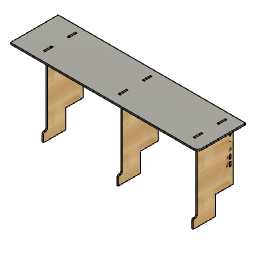
Overall_proto_v3 (Autodesk Fusion 360 design; units mm, degrees)
Autodesk Fusion 360 part; units mm, degrees
sketch "Sketch1" plane through (0, 0, 0) normal (0, 0, 1) x (1, 0, 0)
  line L0 (-1175, 300) -> (1175, 300)
  line L1 (1175, 300) -> (1175, -300)
  line L2 (1175, -300) -> (-1175, -300)
  line L3 (-1175, -300) -> (-1175, 300)
  line L4 (-1175, 300) -> (1175, -300) construction
  line L5 (1175, 300) -> (-1175, -300) construction
  dimension "d5" = 2350
  dimension "d6" = 600
  constraint perpendicular L0 L1
  constraint parallel L0 L2
  constraint parallel L1 L3
  constraint horizontal L0
  constraint coincident L4 origin
  constraint coincident L5 origin
  measures "d5" distance of L1.end L2.end
  measures "d6" distance of L0.end L1.end
extrude "Extrude1" add sketch "Sketch1" along normal blind 18 makes body 1
fillet "Fillet1" radius 50 1 edges at (1175, -300, 9) on bodies 1
sketch "Sketch2" plane through (0, 0, 18) normal (0, 0, 1) x (-1, 0, 0)
  arc A0 (-1125, 300) -> (-1175, 250) centre (-1125, 250) ccw
  line L0 (-1175, 250) -> (-1175, -300)
  line L1 (-1175, -300) -> (1175, -300)
  line L2 (1175, -300) -> (1175, 300)
  line L3 (1175, 300) -> (-1125, 300)
  line L4 (-61, -120) -> (-79, -120)
  line L5 (-79, -120) -> (-79, -220)
  line L6 (-79, -220) -> (-61, -220)
  line L7 (-61, -220) -> (-61, -120)
  line L8 (-61, -120) -> (-79, -220) construction
  line L9 (-79, -120) -> (-61, -220) construction
  point P0 (-70, -170)
  dimension "d10" = 18
  dimension "d11" = 100
  dimension "d12" = 80
  dimension "d23" = 70
  constraint perpendicular L4 L5
  constraint parallel L4 L6
  constraint parallel L5 L7
  constraint horizontal L4
  constraint coincident L8 P0
  constraint coincident L9 P0
  measures "d10" distance of L5.end L6.end
  measures "d11" distance of L4.end L5.end
  measures "d12" distance of L1 L6.end
  measures "d23" horizontal distance of origin P0
extrude "Extrude2" cut sketch "Sketch2" against normal blind 18 contours L4 L5 L6 L7 bodies 1
sketch "Sketch3" plane through (0, 0, 18) normal (0, 0, 1) x (-1, 0, 0)
  line L0 (-79, -120) -> (-61, -120)
  line L1 (-61, -120) -> (-61, -220)
  line L2 (-61, -220) -> (-79, -220)
  line L3 (-79, -220) -> (-79, -120)
  arc A0 (-1125, 300) -> (-1175, 250) centre (-1125, 250) ccw
  line L4 (-1175, 250) -> (-1175, -300)
  line L5 (-1175, -300) -> (1175, -300)
  line L6 (1175, -300) -> (1175, 300)
  line L7 (1175, 300) -> (-1125, 300)
  circle A1 centre (-61, -216.9375) radius 3.0625
  line L8 (-61, -170) -> (-79, -170) construction
  line L9 (-70, -220) -> (-70, -120) construction
  circle A2 centre (-79, -216.9375) radius 3.0625
  line L10 (-61, -120) -> (-79, -120)
  circle A3 centre (-61, -123.0625) radius 3.0625
  circle A4 centre (-79, -123.0625) radius 3.0625
  point P0 (-79, -220)
  point P1 (-79, -120)
  point P2 (-70, -120)
  dimension "d16" = 6.125
  constraint coincident L1 A1.centre
  constraint tangent L2 A1
  constraint midpoint L1 L8.start
  constraint midpoint L3 L8.end
  constraint midpoint L2 L9.start
  constraint midpoint L0 P2
  constraint symmetric L1.end L9 P0
  constraint symmetric A1 L9 A2
  constraint symmetric L1.end L8 L0.end
  constraint symmetric P0 L8 P1
  constraint symmetric A1 L8 A3
  constraint symmetric L8 L9.start P2
  constraint symmetric L8 P0 P1
  constraint symmetric L8 A2 A4
  measures "d16" diameter of A1
extrude "Extrude3" cut sketch "Sketch3" against normal blind 18 contours L3 A4 | L1 A3 | L3 A2 | L1 A1 picked at (-80.1701, -122.9976) picked at (-58.9279, -123.5072) picked at (-80.1701, -217.0024) picked at (-60.4481, -216.0787) bodies 1
pattern_linear "R-Pattern1" count 3 spacing 940 along (1, 0, 0) both ways count 2 spacing 300 along (0, -1, 0) of "Extrude2", "Extrude3"
sketch "Sketch4" plane through (0, 0, 0) normal (1, 0, 0) x (0, 1, 0)
  line L0 (300, -44.3727) -> (-200, -44.3727)
  line L1 (-200, -44.3727) -> (-200, -1008.3727)
  line L2 (-200, -1008.3727) -> (300, -1008.3727)
  line L3 (300, -1008.3727) -> (300, -44.3727)
  line L4 (300, -1008.3727) -> (79, -1008.3727)
  line L5 (79, -1008.3727) -> (79, -768.3727)
  line L6 (79, -768.3727) -> (300, -768.3727)
  line L7 (300, -768.3727) -> (300, -1008.3727)
  line L8 (220, -44.3727) -> (120, -44.3727)
  line L9 (120, -44.3727) -> (120, -26.3727)
  line L10 (120, -26.3727) -> (220, -26.3727)
  line L11 (220, -26.3727) -> (220, -44.3727)
  line L12 (-180, -26.3727) -> (-80, -26.3727)
  line L13 (-180, -44.3727) -> (-180, -26.3727)
  line L14 (-80, -44.3727) -> (-180, -44.3727)
  line L15 (-80, -26.3727) -> (-80, -44.3727)
  dimension "d24" = 964
  dimension "d25" = 500
  dimension "d29" = 240
  dimension "d30" = 221
  dimension "d31" = 100
  dimension "d32" = 18
  dimension "d35" = 80
  dimension "d38" = 300
  dimension "d39" = 0
  constraint horizontal L0
  constraint vertical L1
  constraint horizontal L2
  constraint vertical L3
  constraint horizontal L4
  constraint vertical L5
  constraint horizontal L6
  constraint vertical L7
  constraint horizontal L8
  constraint vertical L9
  constraint horizontal L10
  constraint vertical L11
  constraint coincident L0 L8.start
  measures "d24" distance of L0.start L2.end
  measures "d25" distance of L0.start L0.end
  measures "d29" distance of L2.end L6.end
  measures "d30" distance of L2.end L4.end
  measures "d31" distance of L8.start L8.end
  measures "d32" distance of L8.start L10.end
  measures "d35" distance of L3 L8.start
extrude "Extrude4" add sketch "Sketch4" along normal blind 18 separate body contours L0 L1 L2 L3 L5 L6 L8 L14 | L0 L8 L9 L10 L11 | L0 L12 L13 L14 L15 makes body 2
sketch "Sketch5" plane through (0, 0, 0) normal (-1, 0, 0) x (0, -1, 0)
  line L0 (200, -44.3727) -> (180, -44.3727)
  line L1 (180, -44.3727) -> (180, -26.3727)
  line L2 (180, -26.3727) -> (80, -26.3727)
  line L3 (80, -26.3727) -> (80, -44.3727)
  line L4 (80, -44.3727) -> (-120, -44.3727)
  line L5 (-120, -44.3727) -> (-120, -26.3727)
  line L6 (-120, -26.3727) -> (-220, -26.3727)
  line L7 (-220, -26.3727) -> (-220, -44.3727)
  line L8 (-220, -44.3727) -> (-300, -44.3727)
  line L9 (-300, -44.3727) -> (-300, -768.3727)
  line L10 (-300, -768.3727) -> (-79, -768.3727)
  line L11 (-79, -768.3727) -> (-79, -1008.3727)
  line L12 (-79, -1008.3727) -> (200, -1008.3727)
  line L13 (200, -1008.3727) -> (200, -44.3727)
  circle A0 centre (-223.0625, -44.3727) radius 3.0625
  circle A1 centre (-116.9375, -44.3727) radius 3.0625
  circle A2 centre (183.0625, -44.3727) radius 3.0625
  circle A3 centre (76.9375, -44.3727) radius 3.0625
  point P0 (-113.875, -44.3727)
  point P1 (186.125, -44.3727)
  point P2 (180, -44.3727)
  point P3 (80, -44.3727)
  dimension "d42" = 6.125
  dimension "d45" = 106.125
  dimension "d46" = 0
  dimension "d49" = 300
  dimension "d50" = 0
  constraint coincident L7.end A0
  measures "d42" diameter of A0
extrude "Extrude5" cut sketch "Sketch5" against normal blind 18 contours L0 A2 | L4 A3 | L8 A0 | L4 A1 picked at (183.1388, -45.3906) picked at (76.8612, -45.3906) picked at (-223.1388, -45.3906) picked at (-117.0138, -45.3906) bodies 2
fillet "Fillet2" radius 6.125 4 edges at (9, 220, -26.3727) (9, 120, -26.3727) (9, -180, -26.3727) (9, -80, -26.3727) on bodies 2
sketch "Sketch6" plane through (0, 0, 0) normal (-1, 0, 0) x (0, -1, 0)
  arc A0 (86.125, -26.3727) -> (80, -32.4977) centre (86.125, -32.4977) ccw
  line L0 (80, -32.4977) -> (80, -44.3727)
  arc A1 (73.875, -44.3727) -> (80, -44.3727) centre (76.9375, -44.3727) ccw
  line L1 (73.875, -44.3727) -> (-113.875, -44.3727)
  arc A2 (-120, -44.3727) -> (-113.875, -44.3727) centre (-116.9375, -44.3727) ccw
  line L2 (-120, -44.3727) -> (-120, -32.4977)
  arc A3 (-120, -32.4977) -> (-126.125, -26.3727) centre (-126.125, -32.4977) ccw
  line L3 (-126.125, -26.3727) -> (-213.875, -26.3727)
  arc A4 (-213.875, -26.3727) -> (-220, -32.4977) centre (-213.875, -32.4977) ccw
  line L4 (-220, -32.4977) -> (-220, -44.3727)
  arc A5 (-226.125, -44.3727) -> (-220, -44.3727) centre (-223.0625, -44.3727) ccw
  line L5 (-226.125, -44.3727) -> (-300, -44.3727)
  line L6 (-300, -44.3727) -> (-300, -768.3727)
  line L7 (-300, -768.3727) -> (-79, -768.3727)
  line L8 (-79, -768.3727) -> (-79, -1008.3727)
  line L9 (-79, -1008.3727) -> (200, -1008.3727)
  line L10 (200, -1008.3727) -> (200, -44.3727)
  line L11 (200, -44.3727) -> (186.125, -44.3727)
  arc A6 (180, -44.3727) -> (186.125, -44.3727) centre (183.0625, -44.3727) ccw
  line L12 (180, -44.3727) -> (180, -32.4977)
  arc A7 (180, -32.4977) -> (173.875, -26.3727) centre (173.875, -32.4977) ccw
  line L13 (173.875, -26.3727) -> (86.125, -26.3727)
  circle A8 centre (-79, -771.4352) radius 3.0625
  dimension "d54" = 6.125
  constraint coincident L7.end A8
  measures "d54" diameter of A8
extrude "Extrude6" cut sketch "Sketch6" against normal blind 18 contours L8 A8 picked at (-77.1359, -770.6096) bodies 2
sketch "Sketch7" plane through (18, 0, 0) normal (1, 0, 0) x (0, 1, 0)
  arc A0 (79, -768.3727) -> (79, -774.4977) centre (79, -771.4352) ccw
  line L0 (79, -768.3727) -> (300, -768.3727)
  line L1 (300, -768.3727) -> (300, -44.3727)
  line L2 (300, -44.3727) -> (226.125, -44.3727)
  arc A1 (220, -44.3727) -> (226.125, -44.3727) centre (223.0625, -44.3727) ccw
  line L3 (220, -44.3727) -> (220, -32.4977)
  arc A2 (220, -32.4977) -> (213.875, -26.3727) centre (213.875, -32.4977) ccw
  line L4 (213.875, -26.3727) -> (126.125, -26.3727)
  arc A3 (126.125, -26.3727) -> (120, -32.4977) centre (126.125, -32.4977) ccw
  line L5 (120, -32.4977) -> (120, -44.3727)
  arc A4 (113.875, -44.3727) -> (120, -44.3727) centre (116.9375, -44.3727) ccw
  line L6 (113.875, -44.3727) -> (-73.875, -44.3727)
  arc A5 (-80, -44.3727) -> (-73.875, -44.3727) centre (-76.9375, -44.3727) ccw
  line L7 (-80, -44.3727) -> (-80, -32.4977)
  arc A6 (-80, -32.4977) -> (-86.125, -26.3727) centre (-86.125, -32.4977) ccw
  line L8 (-86.125, -26.3727) -> (-173.875, -26.3727)
  arc A7 (-173.875, -26.3727) -> (-180, -32.4977) centre (-173.875, -32.4977) ccw
  line L9 (-180, -32.4977) -> (-180, -44.3727)
  arc A8 (-186.125, -44.3727) -> (-180, -44.3727) centre (-183.0625, -44.3727) ccw
  line L10 (-186.125, -44.3727) -> (-200, -44.3727)
  line L11 (-200, -44.3727) -> (-200, -1008.3727)
  line L12 (-200, -1008.3727) -> (79, -1008.3727)
  line L13 (79, -1008.3727) -> (79, -774.4977)
  line L14 (-200, -150) -> (-170, -150)
  line L15 (-150, -170) -> (-150, -880)
  line L16 (-170, -900) -> (-200, -900)
  line L17 (-200, -900) -> (-200, -150)
  arc A9 (-150, -170) -> (-170, -150) centre (-170, -170) ccw
  arc A10 (-170, -900) -> (-150, -880) centre (-170, -880) ccw
  dimension "d57" = 20
  constraint horizontal L14
  constraint vertical L15
  constraint horizontal L16
  constraint vertical L17
  constraint coincident L11 L14.start
  constraint tangent L14 A9
  constraint tangent L15 A9
  constraint tangent L15 A10
  constraint tangent L16 A10
  constraint equal A9 A10
  measures "d57" radius of A9
extrude "Extrude7" cut sketch "Sketch7" against normal blind 18 contours L11 L14 L15 L16 L17 A9 A10 bodies 2
sketch "Sketch8" plane through (18, 0, 0) normal (1, 0, 0) x (0, 1, 0)
  line L0 (-200, -150) -> (-170, -150)
  arc A0 (-150, -170) -> (-170, -150) centre (-170, -170) ccw
  line L1 (-150, -170) -> (-150, -880)
  arc A1 (-170, -900) -> (-150, -880) centre (-170, -880) ccw
  line L2 (-170, -900) -> (-200, -900)
  line L3 (-200, -900) -> (-200, -1008.3727)
  line L4 (-200, -1008.3727) -> (79, -1008.3727)
  line L5 (79, -1008.3727) -> (79, -774.4977)
  arc A2 (79, -768.3727) -> (79, -774.4977) centre (79, -771.4352) ccw
  line L6 (79, -768.3727) -> (300, -768.3727)
  line L7 (300, -768.3727) -> (300, -44.3727)
  line L8 (300, -44.3727) -> (226.125, -44.3727)
  arc A3 (220, -32.4977) -> (213.875, -26.3727) centre (213.875, -32.4977) ccw
  line L9 (213.875, -26.3727) -> (126.125, -26.3727)
  arc A4 (126.125, -26.3727) -> (120, -32.4977) centre (126.125, -32.4977) ccw
  line L10 (120, -32.4977) -> (120, -44.3727)
  arc A5 (113.875, -44.3727) -> (120, -44.3727) centre (116.9375, -44.3727) ccw
  line L11 (113.875, -44.3727) -> (-73.875, -44.3727)
  arc A6 (-80, -44.3727) -> (-73.875, -44.3727) centre (-76.9375, -44.3727) ccw
  line L12 (-80, -44.3727) -> (-80, -32.4977)
  arc A7 (-80, -32.4977) -> (-86.125, -26.3727) centre (-86.125, -32.4977) ccw
  line L13 (-86.125, -26.3727) -> (-173.875, -26.3727)
  arc A8 (-173.875, -26.3727) -> (-180, -32.4977) centre (-173.875, -32.4977) ccw
  line L14 (-180, -32.4977) -> (-180, -44.3727)
  arc A9 (-186.125, -44.3727) -> (-180, -44.3727) centre (-183.0625, -44.3727) ccw
  line L15 (-186.125, -44.3727) -> (-200, -44.3727)
  line L16 (-200, -44.3727) -> (-200, -150)
  line L17 (273, -94.3727) -> (273, -144.3727)
  circle A10 centre (258.0625, -144.3727) radius 3.0625
  line L18 (255, -94.3727) -> (273, -94.3727)
  line L19 (273, -144.3727) -> (255, -144.3727)
  line L20 (255, -144.3727) -> (255, -94.3727)
  circle A11 centre (269.9375, -144.3727) radius 3.0625
  circle A12 centre (269.9375, -94.3727) radius 3.0625
  circle A13 centre (258.0625, -94.3727) radius 3.0625
  line L21 (255, -427.706) -> (273, -427.706)
  line L22 (273, -427.706) -> (273, -477.706)
  circle A14 centre (269.9375, -477.706) radius 3.0625
  line L23 (255, -477.706) -> (255, -427.706)
  circle A15 centre (258.0625, -427.706) radius 3.0625
  circle A16 centre (258.0625, -477.706) radius 3.0625
  line L24 (273, -477.706) -> (255, -477.706)
  circle A17 centre (269.9375, -427.706) radius 3.0625
  line L25 (264, -144.3727) -> (264, -427.706) construction
  circle A18 centre (264, -286.0393) radius 2.5
  dimension "d78" = 18
  dimension "d79" = 6.125
  dimension "d80" = 27
  dimension "d81" = 50
  dimension "d84" = 0
  dimension "d85" = -333.3333
  dimension "d86" = 5
  constraint tangent L20 A13
  constraint tangent A10 L20
  constraint tangent L17 A12
  constraint tangent L17 A11
  constraint coincident L18 A13.centre
  constraint coincident L18 A12.centre
  constraint coincident A10.centre L19
  constraint coincident A11.centre L19
  constraint equal A12 A13
  constraint equal A10 A12
  constraint equal A10 A11
  constraint midpoint L19 L25.start
  constraint midpoint L21 L25.end
  constraint midpoint L25 A18.centre
  measures "d78" distance of L17 L20
  measures "d79" diameter of A13
  measures "d80" distance of L7 L17
  measures "d81" distance of L8 L18
  measures "d86" diameter of A18
extrude "Extrude8" cut sketch "Sketch8" against normal blind 18 bodies 2
pattern_linear "R-Pattern2" count 2 spacing 80 along (0, 0, -1) of "Extrude8"
fillet "Fillet3" radius 20 2 edges at (9, -200, -900) (9, -200, -150) on bodies 2
copy_body "Body->Comp1" bodies 1 removing the originals makes body 3 in component "btm_sheet"
copy_body "Body->Comp2" bodies 2 removing the originals makes body 4 in component "stand"
sketch "Sketch9" plane through (0, 0, 0) normal (0, 1, 0) x (1, 0, 0)
  line L0 (74.3329, 269.9769) -> (-901.6671, 269.9769)
  line L1 (-901.6671, 269.9769) -> (-901.6671, 653.3103)
  line L2 (-901.6671, 653.3103) -> (74.3329, 653.3103)
  line L3 (74.3329, 653.3103) -> (74.3329, 269.9769)
  line L4 (74.3329, 319.9769) -> (56.3329, 319.9769)
  line L5 (56.3329, 319.9769) -> (56.3329, 603.3103)
  line L6 (56.3329, 603.3103) -> (74.3329, 603.3103)
  line L7 (74.3329, 603.3103) -> (74.3329, 319.9769)
  circle A0 centre (56.3329, 323.0394) radius 3.0625
  circle A1 centre (56.3329, 600.2478) radius 3.0625
  line L8 (-413.6671, 269.9769) -> (-413.6671, 653.3103) construction
  line L9 (56.3329, 529.1436) -> (56.3329, 494.1436)
  circle A2 centre (-883.6671, 323.0394) radius 3.0625
  line L10 (-901.6671, 603.3103) -> (-901.6671, 319.9769)
  line L11 (-883.6671, 603.3103) -> (-901.6671, 603.3103)
  circle A3 centre (-883.6671, 600.2478) radius 3.0625
  line L12 (-883.6671, 319.9769) -> (-883.6671, 603.3103)
  line L13 (-901.6671, 319.9769) -> (-883.6671, 319.9769)
  line L14 (-883.6671, 529.1436) -> (-883.6671, 494.1436)
  point P0 (-3.6671, 511.6436)
  dimension "d122" = 976
  dimension "d123" = 383.3333
  dimension "d124" = 283.3333
  dimension "d125" = 18
  dimension "d126" = 6.125
  dimension "d127" = 6.125
  constraint horizontal L0
  constraint vertical L1
  constraint horizontal L2
  constraint vertical L3
  constraint horizontal L4
  constraint vertical L5
  constraint horizontal L6
  constraint coincident L3 L4.start
  constraint coincident L4.end A0
  constraint coincident L5.end A1
  constraint midpoint L0 L8.start
  constraint midpoint L2 L8.end
  constraint vertical L9
  constraint coincident L5 L9.end
  constraint symmetric L4.start L8 L10.end
  constraint symmetric L4.end L8 L12.start
  constraint symmetric L5.end L8 L11.start
  constraint symmetric L6.end L8 L10.start
  constraint symmetric A0 L8 A2
  constraint symmetric A1 L8 A3
  constraint symmetric L8 L9.end L14.end
  constraint symmetric L8 L9.start L14.start
  measures "d122" distance of L0.start L0.end
  measures "d123" distance of L0 L2
  measures "d124" distance of L4.start L6.end
  measures "d125" distance of L4.start L4.end
  measures "d126" diameter of A0
  measures "d127" diameter of A1
extrude "Extrude9" add sketch "Sketch9" along normal blind 18 separate body contours L0 L1 L2 L3 L4 L5 L6 A0 A1 L9 A2 L11 A3 L12 L13 L14 makes body 5
fillet "Fillet4" radius 6.125 8 edges at (-901.6671, 9, -653.3103) (-901.6671, 9, -603.3103) (-901.6671, 9, -319.9769) (-901.6671, 9, -269.9769) (74.3329, 9, -319.9769) (74.3329, 9, -269.9769) (74.3329, 9, -603.3103) (74.3329, 9, -653.3103) on bodies 5
sketch "Sketch10" plane through (0, 18, 0) normal (0, 1, 0) x (-1, 0, 0)
  arc A0 (-74.3329, -647.1853) -> (-68.2079, -653.3103) centre (-68.2079, -647.1853) ccw
  line L0 (-68.2079, -653.3103) -> (895.5421, -653.3103)
  arc A1 (895.5421, -653.3103) -> (901.6671, -647.1853) centre (895.5421, -647.1853) ccw
  line L1 (901.6671, -647.1853) -> (901.6671, -609.4353)
  arc A2 (901.6671, -609.4353) -> (895.5421, -603.3103) centre (895.5421, -609.4353) ccw
  line L2 (895.5421, -603.3103) -> (883.6671, -603.3103)
  arc A3 (883.6671, -597.1853) -> (883.6671, -603.3103) centre (883.6671, -600.2478) ccw
  line L3 (883.6671, -597.1853) -> (883.6671, -326.1019)
  arc A4 (883.6671, -319.9769) -> (883.6671, -326.1019) centre (883.6671, -323.0394) ccw
  line L4 (883.6671, -319.9769) -> (895.5421, -319.9769)
  arc A5 (895.5421, -319.9769) -> (901.6671, -313.8519) centre (895.5421, -313.8519) ccw
  line L5 (901.6671, -313.8519) -> (901.6671, -276.1019)
  arc A6 (901.6671, -276.1019) -> (895.5421, -269.9769) centre (895.5421, -276.1019) ccw
  line L6 (895.5421, -269.9769) -> (-68.2079, -269.9769)
  arc A7 (-68.2079, -269.9769) -> (-74.3329, -276.1019) centre (-68.2079, -276.1019) ccw
  line L7 (-74.3329, -276.1019) -> (-74.3329, -313.8519)
  arc A8 (-74.3329, -313.8519) -> (-68.2079, -319.9769) centre (-68.2079, -313.8519) ccw
  line L8 (-68.2079, -319.9769) -> (-56.3329, -319.9769)
  arc A9 (-56.3329, -326.1019) -> (-56.3329, -319.9769) centre (-56.3329, -323.0394) ccw
  line L9 (-56.3329, -326.1019) -> (-56.3329, -597.1853)
  arc A10 (-56.3329, -603.3103) -> (-56.3329, -597.1853) centre (-56.3329, -600.2478) ccw
  line L10 (-56.3329, -603.3103) -> (-68.2079, -603.3103)
  arc A11 (-68.2079, -603.3103) -> (-74.3329, -609.4353) centre (-68.2079, -609.4353) ccw
  line L11 (-74.3329, -609.4353) -> (-74.3329, -647.1853)
  line L12 (413.6671, -269.9769) -> (413.6671, -653.3103) construction
  line L13 (-56.3329, -461.6436) -> (883.6671, -461.6436) construction
  circle A12 centre (-47.5329, -461.6436) radius 11
  circle A13 centre (874.8671, -461.6436) radius 11
  point P0 (883.6671, -461.6436)
  dimension "d139" = 22
  dimension "d140" = 8.8
  constraint midpoint L6 L12.start
  constraint midpoint L0 L12.end
  constraint midpoint L9 L13.start
  constraint midpoint L3 P0
  constraint coincident L13 A12.centre
  constraint symmetric L12 L13.start P0
  constraint symmetric L12 A12 A13
  measures "d139" diameter of A12
  measures "d140" distance of L9 A12.centre
extrude "Extrude10" cut sketch "Sketch10" against normal blind 15 contours L9 A12 | L3 A13 picked at (-48.0122, -458.1862) picked at (869.5556, -460.5814) bodies 5
copy_body "Body->Comp3" bodies 5 removing the originals makes body 6 in component "rear_wall"
copy_body "CopyPasteBodies1" bodies 4 body 4 seen with x (1, 0, 0) y (0, 1, 0) z (0, 0, 1) at (56.3329, -255, -175.6043) makes body 7
move_body "Move1" bodies 7 to x (1, 0, 0) y (0, 1, 0) z (0, 0, 1) at (-940, 0, 0)
copy_body "CopyPasteBodies2" bodies 7 makes body 8
move_body "Move2" bodies 8 to x (1, 0, 0) y (0, 1, 0) z (0, 0, 1) at (1880, 0, 0)
component "btm_sheet" placed x (1, 0, 0) y (0, 1, 0) z (0, 0, 1) at (-4.6671, -255, -219.9769)
component "stand" placed x (1, 0, 0) y (0, 1, 0) z (0, 0, 1) at (56.3329, -255, -175.6043)
component "rear_wall" placed x (1, 0, 0) y (0, 1, 0) z (0, 0, 1) at (0, 0, 0)
equation "table_height = 1000 mm" comment "Высота верстака"
equation "table_length = 2350 mm" comment "Длина верстака"
equation "table_depth = 600 mm" comment "Ширина верстака"
equation "sheet_thickness = 18 mm" comment "Толщина фанеры"
equation "d5 = table_length"
equation "d6 = table_depth"
equation "d7 = sheet_thickness"
equation "d10 = sheet_thickness"
equation "d11 = notch_length"
equation "d12 = notch_gap"
equation "d13 = -sheet_thickness"
equation "mill_diam = 6.125 mm" comment "диаметр фрезы для фанеры"
equation "d16 = mill_diam"
equation "d17 = -sheet_thickness"
equation "d21 = table_length / 2.5"
equation "d22 = -table_depth / 2"
equation "d24 = table_height - 2 * sheet_thickness"
equation "d25 = table_depth - leg_offset"
equation "leg_offset = 100 mm"
equation "box_depth = 221 mm" comment "Глубина короба сбоку"
equation "box_height = 240 mm" comment "Высота ебучего короба"
equation "d29 = box_height"
equation "d30 = box_depth"
equation "d31 = notch_length"
equation "d32 = sheet_thickness"
equation "notch_gap = 80 mm" comment "Отступ от шипа до края"
equation "notch_length = 100 mm" comment "Ширина шипа"
equation "d35 = notch_gap"
equation "d38 = table_depth / 2"
equation "d40 = sheet_thickness"
equation "d42 = mill_diam"
equation "d45 = notch_length + mill_diam"
equation "d49 = table_depth / 2"
equation "d51 = -sheet_thickness"
equation "d53 = mill_diam"
equation "d54 = mill_diam"
equation "d55 = -sheet_thickness"
equation "d58 = -sheet_thickness"
equation "d78 = sheet_thickness"
equation "d80 = sheet_thickness * 1.5"
equation "d81 = table_height / 20"
equation "d85 = table_height / -3"
equation "d87 = -sheet_thickness"
equation "d91 = notch_gap"
equation "d111 = -mill_diam / 2"
equation "d122 = table_length / 2.5 + 2 * sheet_thickness"
equation "d123 = notch_length / 2 + table_height / 3"
equation "d124 = table_height / 3 - notch_length / 2"
equation "d125 = sheet_thickness"
equation "d126 = mill_diam"
equation "d127 = mill_diam"
equation "d136 = sheet_thickness"
equation "d138 = mill_diam"
equation "d143 = mill_diam / 2"
named bodies: "btm_sheet", "stand", "rear_wall", "stand (1)"
